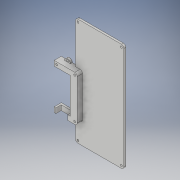
# Autodesk Inventor part: PhoneCover
Saved by Autodesk Inventor 2019 (Build 230136000, 136)
## iProperties
Created: 2019-01-25
Part Number: PhoneCover
Material: Generic
Document SubType Name: Modeling
Designer: garretthagen21
Density: 1 g/cm^3
Appearance: Default
Author: garretthagen21
Autodesk Inventor part; units mm, degrees
ref_plane "YZ Plane" through (0, 0, 0) normal (1, 0, 0) x (0, 1, 0)
ref_plane "XZ Plane" through (0, 0, 0) normal (0, 1, 0) x (-1, 0, 0)
ref_plane "XY Plane" through (0, 0, 0) normal (0, 0, 1) x (1, 0, 0)
sketch "Sketch1" plane through (0, 0, 0) normal (0, 0, 1) x (1, 0, 0)
  line L0 (7.2667, 4.052) -> (-48.1053, 4.052)
  line L1 (-51.2803, 0.877) -> (-51.2803, -50.05)
  line L2 (-51.2803, -107.708) -> (-51.2803, -129.933)
  line L3 (-48.1053, -133.108) -> (7.2667, -133.108)
  line L4 (10.4417, -129.933) -> (10.4417, 0.877)
  line L5 (-51.2803, -101.358) -> (-51.2803, -56.4)
  line L6 (-71.8543, -50.05) -> (-71.8543, -56.4)
  line L7 (-71.8543, -56.4) -> (-51.2803, -56.4)
  line L8 (-51.2803, -107.708) -> (-71.8543, -107.708)
  line L9 (-71.8543, -107.708) -> (-71.8543, -101.358)
  line L10 (-71.8543, -101.358) -> (-51.2803, -101.358)
  arc A0 (-48.1053, 4.052) -> (-51.2803, 0.877) centre (-48.1053, 0.877) ccw
  arc A1 (10.4417, 0.877) -> (7.2667, 4.052) centre (7.2667, 0.877) ccw
  arc A2 (-51.2803, -129.933) -> (-48.1053, -133.108) centre (-48.1053, -129.933) ccw
  arc A3 (7.2667, -133.108) -> (10.4417, -129.933) centre (7.2667, -129.933) ccw
  arc A4 (-57.7573, -50.05) -> (-65.3773, -50.05) centre (-61.5673, -50.05) ccw
  line L11 (-51.2803, -50.05) -> (-57.7573, -50.05)
  line L12 (-65.3773, -50.05) -> (-71.8543, -50.05)
  point P0 (0, 0)
  point P1 (10.4417, 4.052)
  point P2 (-51.2803, 4.052)
  point P3 (-51.2803, -133.108)
  point P4 (10.4417, -133.108)
  dimension "d0" = 61.722
  dimension "d1" = 54.102
  dimension "d4" = 25.4
  dimension "d22" = 20.574
  dimension "d23" = 6.35
  dimension "d24" = 6.35
  dimension "d42" = 137.16
  dimension "d50" = 3.175
  dimension "d53" = 7.62
  constraints: 26 end point, 10 point on circle, 10 point on line, 8 tangent, 5 centre point, 5 perpendicular, 3 equal radius, 3 horizontal, 3 vertical, 2 parallel
  measures "d0" distance of point (10.442, 4.052) point (-51.28, 4.052)
  measures "d1" distance of point (-51.28, 4.052) L1.end
  measures "d4" distance of L2.start point (-51.28, -133.108)
  measures "d22" distance of L1.end L6.start
  measures "d23" distance of L6.start L6.end
  measures "d24" distance of L8.end L9.end
  measures "d42" distance between parallel lines of L3 L0
  measures "d50" radius of A0
  measures "d53" diameter of A4
extrude "Phone Cover" add sketch "Sketch1" along normal blind 2.54
sketch "Sketch2" plane through (0, 0, 2.54) normal (0, 0, 1) x (1, 0, 0)
  line L0 (7.2667, 4.052) -> (-48.1053, 4.052) projected
  line L1 (-51.2803, 0.877) -> (-51.2803, -50.05) projected
  line L2 (10.4417, -129.933) -> (10.4417, 0.877) projected
  line L3 (-48.1053, -133.108) -> (7.2667, -133.108) projected
  point P0 (0, 0)
  point P1 (-48.1053, 0.877)
  point P2 (10.4417, 4.052)
  point P3 (-51.2803, 4.052)
  point P4 (-51.2803, -133.108)
  point P5 (7.2667, 0.877)
  point P6 (10.4417, -133.108)
  point P7 (-48.1053, -129.933)
  point P8 (7.2667, -129.933)
  dimension "d7" = 3.175
  dimension "d8" = 3.175
  dimension "d9" = 3.175
  dimension "d10" = 3.175
  dimension "d43" = 3.175
  dimension "d44" = 3.175
  dimension "d45" = 3.175
  dimension "d46" = 3.175
  measures "d7" distance from line of L0 point (-48.105, 0.877)
  measures "d8" distance from line of L1 point (-48.105, 0.877)
  measures "d9" distance from line of L2 point (7.267, 0.877)
  measures "d10" distance from line of L3 point (-48.105, -129.933)
  measures "d43" distance from line of L0 point (7.267, 0.877)
  measures "d44" distance from line of point (-48.105, -129.933) L1
  measures "d45" distance from line of point (7.267, -129.933) L2
  measures "d46" distance from line of point (7.267, -129.933) L3
hole "Phone Holes" at (-48.1053, 0.877, 2.54) at (7.2667, 0.877, 2.54) at (-48.1053, -129.933, 2.54) at (7.2667, -129.933, 2.54) direction (0, 0, -1) diameter 2.54 depth 25.4 tip angle 118
sketch "Sketch3" plane through (0, 0, 2.54) normal (0, 0, 1) x (1, 0, 0)
  line L0 (-51.2803, -107.708) -> (-45.5653, -107.708)
  line L1 (-51.2803, -50.05) -> (-45.5653, -50.05)
  line L2 (-42.3903, -53.225) -> (-42.3903, -104.533)
  line L3 (-51.2803, -50.05) -> (-71.8543, -50.05) projected
  line L4 (-71.8543, -56.4) -> (-51.2803, -56.4) projected
  line L5 (-51.2803, -56.4) -> (-71.8543, -56.4)
  line L6 (-71.8543, -56.4) -> (-71.8543, -50.05)
  line L7 (-51.2803, -101.358) -> (-71.8543, -101.358) projected
  line L8 (-51.2803, -101.358) -> (-54.4553, -101.358)
  line L9 (-71.8543, -107.708) -> (-51.2803, -107.708) projected
  line L10 (-54.4553, -107.708) -> (-51.2803, -107.708)
  line L11 (-54.4553, -101.358) -> (-54.4553, -107.708)
  line L12 (-71.8543, -101.358) -> (-69.5683, -101.358)
  line L13 (-69.5683, -101.358) -> (-69.5683, -107.708)
  line L14 (-69.5683, -107.708) -> (-71.8543, -107.708)
  line L15 (-71.8543, -107.708) -> (-71.8543, -101.358)
  line L16 (-51.2803, -56.4) -> (-51.2803, -101.358)
  arc A0 (-42.3903, -53.225) -> (-45.5653, -50.05) centre (-45.5653, -53.225) ccw
  arc A1 (-45.5653, -107.708) -> (-42.3903, -104.533) centre (-45.5653, -104.533) ccw
  arc A2 (-57.7573, -50.05) -> (-65.3773, -50.05) centre (-61.5673, -50.05) ccw
  line L17 (-71.8543, -50.05) -> (-65.3773, -50.05)
  line L18 (-57.7573, -50.05) -> (-51.2803, -50.05)
  point P0 (0, 0)
  point P1 (-51.2803, 4.052)
  point P2 (-51.2803, -133.108)
  point P3 (-42.3903, -107.708)
  point P4 (-42.3903, -50.05)
  dimension "d25" = 2.286
  dimension "d26" = 3.175
  dimension "d33" = 8.89
  dimension "d49" = 3.175
  dimension "d52" = 7.62
  constraints: 30 end point, 7 point on line, 6 point on circle, 4 parallel, 4 tangent, 3 centre point, 3 horizontal, 2 perpendicular, 2 vertical, 1 collinear, 1 equal radius
  measures "d25" distance of L13.end L14.end
  measures "d26" distance of L7.start L8.end
  measures "d33" distance between parallel lines of L2 L16
  measures "d49" radius of A0
  measures "d52" diameter of A2
extrude "Scanner Wall" add sketch "Sketch3" along normal blind 6.604 contours L9 L11 L7 L16 L4 L6 L3 L1 A0 L2 A1 L0 | L9 L15 L7 L13
sketch "Sketch4" plane through (0, 0, 9.144) normal (0, 0, 1) x (1, 0, 0)
  line L0 (-45.5653, -50.05) -> (-71.8543, -50.05) projected
  line L1 (-42.3903, -104.533) -> (-42.3903, -53.225) projected
  line L2 (-71.8543, -50.05) -> (-71.8543, -56.4) projected
  line L3 (-54.4553, -107.708) -> (-45.5653, -107.708) projected
  point P0 (0, 0)
  point P1 (-45.5653, -53.225)
  point P2 (-42.3903, -50.05)
  point P3 (-42.3903, -107.708)
  point P4 (-45.5653, -104.533)
  point P5 (-68.6793, -53.225)
  dimension "d29" = 3.175
  dimension "d30" = 3.175
  dimension "d32" = 3.175
  dimension "d41" = 3.175
  dimension "d48" = 3.175
  dimension "d51" = 3.175
  measures "d29" distance from line of point (-45.565, -53.225) L0
  measures "d30" distance from line of point (-45.565, -53.225) L1
  measures "d32" distance from line of point (-45.565, -104.533) L3
  measures "d41" distance from line of L1 point (-45.565, -104.533)
  measures "d48" distance from line of L2 point (-68.679, -53.225)
  measures "d51" distance from line of point (-68.679, -53.225) L0
hole "Scanner Holes" at (-45.5653, -53.225, 9.144) at (-45.5653, -104.533, 9.144) at (-68.6793, -53.225, 9.144) direction (0, 0, -1) diameter 2.54 depth 4.572 tip angle 118
sketch "Sketch5" plane through (0, 0, 2.54) normal (0, 0, 1) x (1, 0, 0)
  line L0 (-65.3773, -50.05) -> (-57.7573, -50.05) projected
  point P0 (0, 0)
  point P1 (-61.5673, -48.526)
  dimension "d54" = 1.524
  measures "d54" distance from line of L0 point (-61.567, -48.526)
hole "Hole3" at (-61.5673, -48.526, 2.54) direction (0, 0, -1) diameter 2.54 depth 8.89 tip angle 118
body "Solid1"
